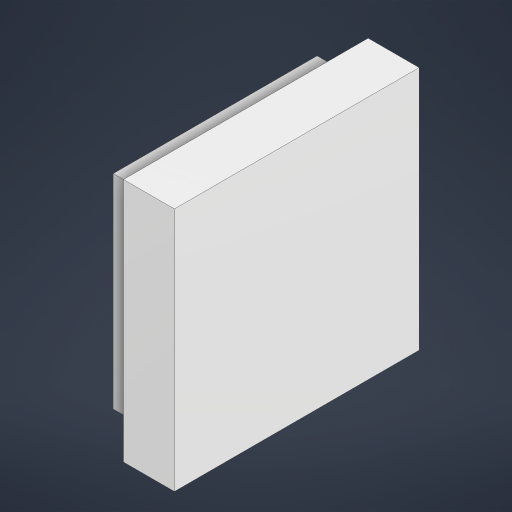
# Autodesk Inventor part: Cuvette_Lid
Saved by Autodesk Inventor 2024.1 (Build 281209000, 209)
## iProperties
Created: 2024-08-12
Part Number: Cuvette_Lid
Material: ABS Plastic
Document SubType Name: Modeling
Designer: Tim Jäger
Density: 1.06 g/cm^3
Appearance: Smooth - White
Author: Tim Jäger
Autodesk Inventor part; units mm, degrees
ref_plane "YZ Plane" through (0, 0, 0) normal (1, 0, 0) x (0, 1, 0)
ref_plane "XZ Plane" through (0, 0, 0) normal (0, 1, 0) x (-1, 0, 0)
ref_plane "XY Plane" through (0, 0, 0) normal (0, 0, 1) x (1, 0, 0)
sketch "Sketch1" plane through (0, 0, 0) normal (1, 0, 0) x (0, 1, 0)
  line L0 (-6, -6) -> (6, -6)
  line L1 (6, -6) -> (6, 6)
  line L2 (6, 6) -> (-6, 6)
  line L3 (-6, 6) -> (-6, -6)
  line L4 (-6, -6) -> (6, 6) construction
  line L5 (6, -6) -> (-6, 6) construction
  point P0 (0, 0)
  dimension "d0" = 12
  dimension "d1" = 12
  constraints: 12 end point, 2 midpoint, 2 parallel, 1 horizontal, 1 perpendicular
  measures "d0" distance of L2.end L1.end
  measures "d1" distance of L1.end L0.end
extrude "Extrusion1" add sketch "Sketch1" along normal blind 2.5
sketch "Sketch2" plane through (0, 0, 0) normal (-1, 0, 0) x (0, 0, 1)
  line L0 (5, -5) -> (-5, -5)
  line L1 (-5, -5) -> (-5, 5)
  line L2 (-5, 5) -> (5, 5)
  line L3 (5, 5) -> (5, -5)
  line L4 (5, -5) -> (-5, 5) construction
  line L5 (-5, -5) -> (5, 5) construction
  point P0 (0, 0)
  dimension "d4" = 10
  dimension "d5" = 10
  constraints: 12 end point, 2 midpoint, 2 parallel, 1 horizontal, 1 perpendicular
  measures "d4" distance of L1.end L2.end
  measures "d5" distance of L0.end L1.end
extrude "Extrusion2" add sketch "Sketch2" along normal blind 1.5
body "Solid1"
